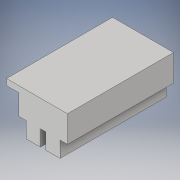
# Autodesk Inventor part: AblakProfil
Saved by Autodesk Inventor 2019 (Build 230136000, 136)
## iProperties
Created: 2022-08-26
Part Number: AblakProfil
Material: Generic
Document SubType Name: Modeling
Designer: laca
Density: 1 g/cm^3
Appearance: Default
Author: laca
Autodesk Inventor part; units mm, degrees
ref_plane "YZ Plane" through (0, 0, 0) normal (1, 0, 0) x (0, 1, 0)
ref_plane "XZ Plane" through (0, 0, 0) normal (0, 1, 0) x (-1, 0, 0)
ref_plane "XY Plane" through (0, 0, 0) normal (0, 0, 1) x (1, 0, 0)
sketch "Sketch1" plane through (0, 0, 0) normal (0, 0, 1) x (1, 0, 0)
  line L0 (0, 0) -> (-92, 0)
  line L1 (-92, 0) -> (-92, 50)
  line L2 (-92, 50) -> (0, 50)
  line L3 (0, 50) -> (0, 0)
  line L4 (-92, 50) -> (-115, 50)
  line L5 (-115, 50) -> (-115, 38.4483)
  line L6 (-115, 38.4483) -> (-92, 38.4483)
  line L7 (-92, 38.4483) -> (-92, 50)
  line L8 (-14, 0) -> (-41, 0)
  line L9 (-41, 0) -> (-41, -30)
  line L10 (-41, -30) -> (-14, -30)
  line L11 (-14, -30) -> (-14, 0)
  line L12 (-78, 0) -> (-51, 0)
  line L13 (-51, 0) -> (-51, -30)
  line L14 (-51, -30) -> (-78, -30)
  line L15 (-78, -30) -> (-78, 0)
  dimension "d0" = 92
  dimension "d1" = 50
  dimension "d2" = 23
  dimension "d3" = 27
  dimension "d4" = 27
  dimension "d5" = 30
  dimension "d6" = 14
  dimension "d7" = 14
  dimension "d8" = 10
  constraints: 32 end point, 8 parallel, 4 horizontal, 4 perpendicular, 3 point on line
  measures "d0" distance of L1.end L2.end
  measures "d1" distance of L0.end L1.end
  measures "d2" distance of L5.end L6.end
  measures "d3" distance of L13.end L14.end
  measures "d4" distance of L9.end L10.end
  measures "d5" distance of L10.end L8.start
  measures "d6" distance between parallel lines of L1 L15
  measures "d7" distance between parallel lines of L3 L11
  measures "d8" distance between parallel lines of L9 L13
extrude "Extrusion1" add sketch "Sketch1" along normal blind 200
equation "\"d4\" = d3"
body "Solid1"
